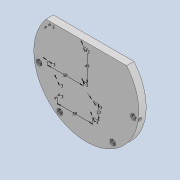
# Autodesk Inventor part: plate_third_floor
Saved by Autodesk Inventor 2020.4 (Build 244396000, 396)
## iProperties
Created: 2021-05-05
Part Number: plate_third_floor
Material: Generic
Document SubType Name: Modeling
Designer: Acer
Density: 1 g/cm^3
Appearance: Default
Author: Acer
Autodesk Inventor part; units mm, degrees
sketch "Sketch1" plane through (0, 0, 0) normal (0, 0, 1) x (1, 0, 0)
  circle A0 centre (0, 0) radius 85.8
  line L0 (-72.5268, -13.7582) -> (-76.3217, -16.8148)
  line L1 (-76.3217, -16.8148) -> (-80.8663, -15.0566)
  line L2 (-80.8663, -15.0566) -> (-81.616, -10.2418)
  line L3 (-81.616, -10.2418) -> (-77.8211, -7.1852)
  line L4 (-77.8211, -7.1852) -> (-73.2765, -8.9434)
  line L5 (-73.2765, -8.9434) -> (-72.5268, -13.7582)
  line L6 (73.2765, -8.9434) -> (77.8211, -7.1852)
  line L7 (77.8211, -7.1852) -> (81.616, -10.2418)
  line L8 (81.616, -10.2418) -> (80.8663, -15.0566)
  line L9 (80.8663, -15.0566) -> (76.3217, -16.8148)
  line L10 (76.3217, -16.8148) -> (72.5268, -13.7582)
  line L11 (72.5268, -13.7582) -> (73.2765, -8.9434)
  line L12 (-77.0714, -12) -> (0, 0) construction
  line L13 (77.0714, -12) -> (0, 0) construction
  line L14 (0, 0) -> (85.8, 0) construction
  line L15 (47.5879, -67.0929) -> (43.5316, -69.793)
  line L16 (47.2777, -62.2299) -> (47.5879, -67.0929)
  line L17 (42.9111, -60.0671) -> (47.2777, -62.2299)
  line L18 (38.8548, -62.7673) -> (42.9111, -60.0671)
  line L19 (39.165, -67.6302) -> (38.8548, -62.7673)
  line L20 (43.5316, -69.793) -> (39.165, -67.6302)
  line L21 (-47.2777, -62.2299) -> (-42.9111, -60.0671)
  line L22 (-42.9111, -60.0671) -> (-38.8548, -62.7673)
  line L23 (-38.8548, -62.7673) -> (-39.165, -67.6302)
  line L24 (-39.165, -67.6302) -> (-43.5316, -69.793)
  line L25 (-43.5316, -69.793) -> (-47.5879, -67.0929)
  line L26 (-47.5879, -67.0929) -> (-47.2777, -62.2299)
  line L27 (-65.8532, 55) -> (65.8532, 55)
  circle A1 centre (77.0714, -12) radius 1.5
  circle A2 centre (43.2214, -64.9301) radius 1.5
  circle A3 centre (-43.2214, -64.9301) radius 1.5
  circle A4 centre (-77.0714, -12) radius 1.5
  dimension "d0" = 171.6
  dimension "d1" = 78
  dimension "d2" = 78
  dimension "d5" = 12
  dimension "d6" = 4.22
  dimension "d7" = 4.22
  dimension "d10" = 12
  dimension "d13" = 47.5
  dimension "d17" = 47.5
  dimension "d19" = 55
  dimension "d81" = 3
  dimension "d82" = 3
  dimension "d83" = 3
  dimension "d84" = 3
  constraints: 56 end point, 5 centre point, 5 coincident, 3 point on circle, 2 horizontal, 2 perpendicular, 54 other
  measures "d0" diameter of A0
  measures "d1" distance of L12.start point (0, 0)
  measures "d2" distance of point (0, 0) L13.start
  measures "d5" distance from line of L14 L13.start
  measures "d6" distance from line of L13.start L11
  measures "d7" distance from line of L5 L12.start
  measures "d10" vertical distance of point (0, 0) L12.start
  measures "d19" distance from line of L27 L12.end
  measures "d81" diameter of A1
  measures "d82" diameter of A2
  measures "d83" diameter of A3
  measures "d84" diameter of A4
extrude "Extrusion1" add sketch "Sketch1" against normal blind 12 contours A0 L27 | A1 | A2 | A3 | A4 picked at (21.9511, 12.3711)
sketch "Sketch2" plane through (0, 0, -12) normal (0, 0, -1) x (-1, 0, 0)
  arc A0 (-65.8532, 55) -> (65.8532, 55) centre (0, 0) ccw projected
  line L0 (65.8532, 55) -> (-65.8532, 55) projected
  line L1 (76.3217, -16.8148) -> (72.5268, -13.7582) projected
  line L2 (72.5268, -13.7582) -> (73.2765, -8.9434) projected
  line L3 (73.2765, -8.9434) -> (77.8211, -7.1852) projected
  line L4 (77.8211, -7.1852) -> (81.616, -10.2418) projected
  line L5 (81.616, -10.2418) -> (80.8663, -15.0566) projected
  line L6 (80.8663, -15.0566) -> (76.3217, -16.8148) projected
  line L7 (-77.8211, -7.1852) -> (-73.2765, -8.9434) projected
  line L8 (-73.2765, -8.9434) -> (-72.5268, -13.7582) projected
  line L9 (-72.5268, -13.7582) -> (-76.3217, -16.8148) projected
  line L10 (-76.3217, -16.8148) -> (-80.8663, -15.0566) projected
  line L11 (-80.8663, -15.0566) -> (-81.616, -10.2418) projected
  line L12 (-81.616, -10.2418) -> (-77.8211, -7.1852) projected
  line L13 (-43.5316, -69.793) -> (-47.5879, -67.0929) projected
  line L14 (-47.5879, -67.0929) -> (-47.2777, -62.2299) projected
  line L15 (-47.2777, -62.2299) -> (-42.9111, -60.0671) projected
  line L16 (-42.9111, -60.0671) -> (-38.8548, -62.7673) projected
  line L17 (-38.8548, -62.7673) -> (-39.165, -67.6302) projected
  line L18 (-39.165, -67.6302) -> (-43.5316, -69.793) projected
  line L19 (42.9111, -60.0671) -> (47.2777, -62.2299) projected
  line L20 (47.2777, -62.2299) -> (47.5879, -67.0929) projected
  line L21 (47.5879, -67.0929) -> (43.5316, -69.793) projected
  line L22 (43.5316, -69.793) -> (39.165, -67.6302) projected
  line L23 (39.165, -67.6302) -> (38.8548, -62.7673) projected
  line L24 (38.8548, -62.7673) -> (42.9111, -60.0671) projected
extrude "Extrusion2" add sketch "Sketch2" against normal blind 4 contours L1 L2 L3 L4 L5 L6 | L7 L8 L9 L10 L11 L12 | L13 L14 L15 L16 L17 L18 | L19 L20 L21 L22 L23 L24
sketch "Sketch3" plane through (80.8663, -15.0566, -8) normal (-0.9881, 0.1538, 0) x (0, 0, 1)
  line L0 (0, 4.8728) -> (0, 0) projected
  line L1 (8, 0) -> (0, 0) projected
  line L2 (8, 4.8728) -> (8, 0) projected
  line L3 (8, 4.8728) -> (0, 4.8728) projected
  circle A0 centre (5, 2.4364) radius 1.5
  point P0 (8, 2.4364)
  dimension "d24" = 3
  dimension "d26" = 5
  dimension "d27" = 2.4364
  constraints: 1 centre point
  measures "d24" diameter of A0
  measures "d26" distance from line of A0.centre L0
  measures "d27" distance from line of A0.centre L1
extrude "Extrusion3" cut sketch "Sketch3" against normal blind 5 contours A0
sketch "Sketch4" plane through (43.5316, -69.793, 0) normal (-0.5541, 0.8324, 0) x (0.8324, 0.5541, 0)
  line L0 (4.8728, 8) -> (0, 8) projected
  line L1 (0, 0) -> (0, 8) projected
  line L2 (4.8728, 0) -> (0, 0) projected
  line L3 (4.8728, 0) -> (4.8728, 8) projected
  circle A0 centre (2.4364, 3) radius 1.5
  point P0 (2.4364, 0)
  dimension "d30" = 3
  dimension "d31" = 5
  dimension "d32" = 2.4364
  constraints: 1 centre point
  measures "d30" diameter of A0
  measures "d31" distance from line of L0 A0.centre
  measures "d32" distance from line of L1 A0.centre
extrude "Extrusion4" cut sketch "Sketch4" against normal blind 5 contours A0
sketch "Sketch5" plane through (-47.5879, -67.0929, 0) normal (0.5541, 0.8324, 0) x (0.8324, -0.5541, 0)
  line L0 (4.8728, 8) -> (0, 8) projected
  line L1 (0, 0) -> (0, 8) projected
  line L2 (4.8728, 0) -> (0, 0) projected
  line L3 (4.8728, 0) -> (4.8728, 8) projected
  circle A0 centre (2.4364, 3) radius 1.5
  point P0 (2.4364, 0)
  dimension "d35" = 3
  dimension "d36" = 2.4364
  dimension "d37" = 5
  constraints: 1 centre point
  measures "d35" diameter of A0
  measures "d36" distance from line of A0.centre L1
  measures "d37" distance from line of A0.centre L0
extrude "Extrusion5" cut sketch "Sketch5" against normal blind 5 contours A0
sketch "Sketch6" plane through (-81.616, -10.2418, 0) normal (0.9881, 0.1538, 0) x (0, 0, -1)
  line L0 (8, -4.8728) -> (8, 0) projected
  line L1 (0, 0) -> (8, 0) projected
  line L2 (0, -4.8728) -> (0, 0) projected
  line L3 (0, -4.8728) -> (8, -4.8728) projected
  circle A0 centre (3, -2.4364) radius 1.5
  point P0 (0, -2.4364)
  dimension "d40" = 3
  dimension "d41" = 2.4364
  dimension "d42" = 5
  constraints: 1 centre point
  measures "d40" diameter of A0
  measures "d41" distance from line of A0.centre L1
  measures "d42" distance from line of L0 A0.centre
extrude "Extrusion6" cut sketch "Sketch6" against normal blind 5 contours A0
ref_plane "Work Plane1" through (82.8425, -15.3643, -8) normal (-0.9881, 0.1538, 0) x (0, 0, 1)
sketch "Sketch7" plane through (82.8425, -15.3643, -8) normal (-0.9881, 0.1538, 0) x (0, 0, 1)
  circle A0 centre (5, 2.4364) radius 1.5 projected
  circle A1 centre (5, 2.4364) radius 2.75
  point P0 (8, 2.4364)
  dimension "d46" = 5.5
  constraints: 1 centre point, 1 coincident
  measures "d46" diameter of A1
extrude "Extrusion7" cut sketch "Sketch7" against normal up to surface contours A0 | A1
ref_plane "Work Plane2" through (44.6398, -71.4579, 0) normal (-0.5541, 0.8324, 0) x (0.8324, 0.5541, 0)
sketch "Sketch8" plane through (44.6398, -71.4579, 0) normal (-0.5541, 0.8324, 0) x (0.8324, 0.5541, 0)
  circle A0 centre (2.4364, 3) radius 1.5 projected
  circle A1 centre (2.4364, 3) radius 2.75
  point P0 (2.4364, 0)
  dimension "d50" = 5.5
  constraints: 1 centre point, 1 coincident
  measures "d50" diameter of A1
extrude "Extrusion8" cut sketch "Sketch8" against normal up to surface contours A0 | A1
ref_plane "Work Plane3" through (-48.6961, -68.7578, 0) normal (0.5541, 0.8324, 0) x (0.8324, -0.5541, 0)
sketch "Sketch9" plane through (-48.6961, -68.7578, 0) normal (0.5541, 0.8324, 0) x (0.8324, -0.5541, 0)
  circle A0 centre (2.4364, 3) radius 1.5 projected
  circle A1 centre (2.4364, 3) radius 2.75
  point P0 (2.4364, 0)
  dimension "d54" = 5.5
  constraints: 1 centre point, 1 coincident
  measures "d54" diameter of A1
extrude "Extrusion9" cut sketch "Sketch9" against normal up to surface contours A0 | A1
ref_plane "Work Plane4" through (-83.5922, -10.5495, 0) normal (0.9881, 0.1538, 0) x (0, 0, -1)
sketch "Sketch10" plane through (-83.5922, -10.5495, 0) normal (0.9881, 0.1538, 0) x (0, 0, -1)
  circle A0 centre (3, -2.4364) radius 1.5 projected
  circle A1 centre (3, -2.4364) radius 2.75
  point P0 (0, -2.4364)
  dimension "d58" = 5.5
  constraints: 1 centre point, 1 coincident
  measures "d58" diameter of A1
extrude "Extrusion10" cut sketch "Sketch10" against normal up to surface contours A0 | A1
sketch "Sketch11" plane through (0, 0, -12) normal (0, 0, -1) x (-1, 0, 0)
  line L0 (75.3409, 34.7165) -> (17.3409, 34.7165) construction
  line L1 (17.3409, 34.7165) -> (17.3409, -14.2835) construction
  line L2 (17.3409, -14.2835) -> (75.3409, -14.2835) construction
  line L3 (75.3409, -14.2835) -> (75.3409, 34.7165) construction
  circle A0 centre (75.3409, 34.7165) radius 1.5
  circle A1 centre (75.3409, -14.2835) radius 1.5
  circle A2 centre (17.3409, 34.7165) radius 1.5
  circle A3 centre (17.3409, -14.2835) radius 1.5
  line L4 (59.7604, -34.3641) -> (1.7604, -34.3641) construction
  line L5 (1.7604, -34.3641) -> (1.7604, -57.3641) construction
  line L6 (1.7604, -57.3641) -> (59.7604, -57.3641) construction
  line L7 (59.7604, -57.3641) -> (59.7604, -34.3641) construction
  circle A4 centre (59.7604, -34.3641) radius 1.5
  circle A5 centre (59.7604, -57.3641) radius 1.5
  circle A6 centre (1.7604, -57.3641) radius 1.5
  circle A7 centre (1.7604, -34.3641) radius 1.5
  dimension "d69" = 58
  dimension "d70" = 49
  dimension "d71" = 3
  dimension "d72" = 3
  dimension "d73" = 3
  dimension "d74" = 3
  dimension "d75" = 58
  dimension "d76" = 23
  dimension "d77" = 3
  dimension "d78" = 3
  dimension "d79" = 3
  dimension "d80" = 3
  constraints: 16 end point, 8 centre point, 8 coincident, 4 parallel, 2 horizontal, 2 perpendicular
  measures "d69" distance of L2.end L1.end
  measures "d70" distance of L1.end L0.end
  measures "d71" diameter of A0
  measures "d72" diameter of A1
  measures "d73" diameter of A2
  measures "d74" diameter of A3
  measures "d75" distance of L6.end L5.end
  measures "d76" distance of L5.end L4.end
  measures "d77" diameter of A4
  measures "d78" diameter of A5
  measures "d79" diameter of A6
  measures "d80" diameter of A7
body "Solid1"
